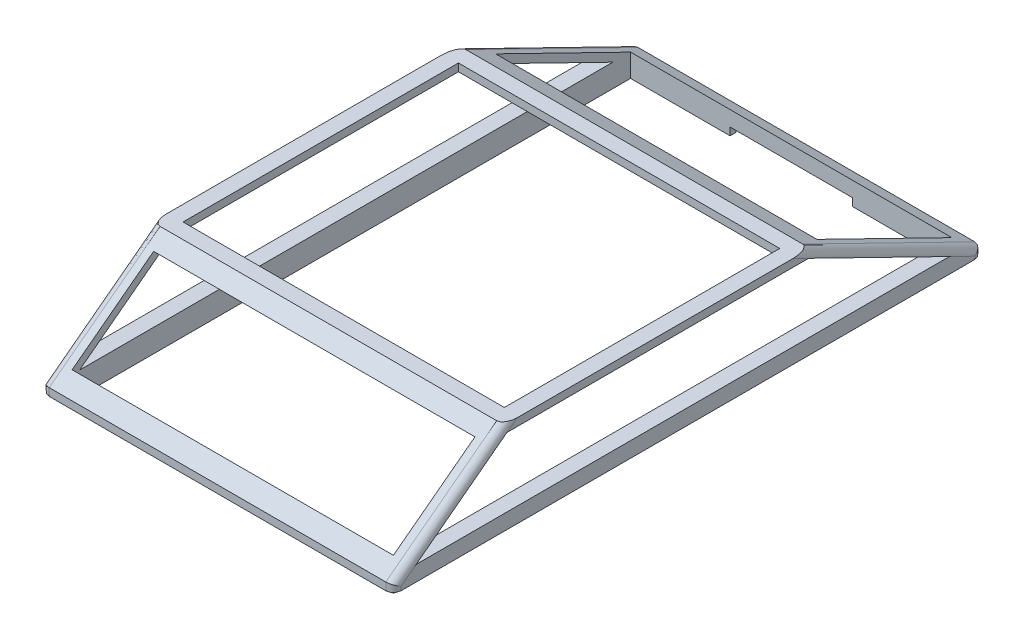
# Autodesk Inventor part: TopLid
Saved by Autodesk Inventor 2023.4 (Build 274418000, 418)
## iProperties
Created: 2026-02-22
Part Number: TopLid
Material: Generic
Document SubType Name: Modeling
Designer: 1017208
Density: 1 g/cm^3
Appearance: Default
Author: 1017208
## iProperties of the stored document TopLid_3DPrint.ipt
Created: 2026-02-22
Part Number: TopLid_3DPrint
Material: Generic
Document SubType Name: Modeling
Designer: 1017208
Density: 1 g/cm^3
Appearance: Default
Author: 1017208
Autodesk Inventor part; units mm, degrees
ref_plane "YZ Plane" through (0, 0, 0) normal (1, 0, 0) x (0, 1, 0)
ref_plane "XZ Plane" through (0, 0, 0) normal (0, 1, 0) x (-1, 0, 0)
ref_plane "XY Plane" through (0, 0, 0) normal (0, 0, 1) x (1, 0, 0)
sketch "Sketch1" plane through (0, 0, 0) normal (0, 1, 0) x (-1, 0, 0)
  line L0 (0, 0) -> (-139.7, 0)
  line L1 (-139.7, 0) -> (-139.7, -238.125)
  line L2 (-139.7, -238.125) -> (0, -238.125)
  line L3 (0, -238.125) -> (0, 0)
  line L4 (-3.175, -3.175) -> (-136.525, -3.175)
  line L5 (-136.525, -3.175) -> (-136.525, -234.95)
  line L6 (-136.525, -234.95) -> (-3.175, -234.95)
  line L7 (-3.175, -234.95) -> (-3.175, -3.175)
  line L8 (0, -238.125) -> (-139.7, -238.125)
  line L9 (-69.85, -238.125) -> (-59.69, -238.125)
  line L10 (-59.69, -238.125) -> (-80.01, -238.125)
  line L11 (-80.01, -234.95) -> (-59.69, -234.95)
  line L12 (-69.85, -238.125) -> (-69.85, -234.95)
  line L13 (-69.85, -238.125) -> (-44.45, -238.125)
  line L14 (-44.45, -238.125) -> (-95.25, -238.125)
  line L15 (-95.25, -238.125) -> (-95.25, -234.95)
  line L16 (-95.25, -234.95) -> (-44.45, -234.95)
  line L17 (-44.45, -234.95) -> (-44.45, -238.125)
  line L18 (-44.45, -238.125) -> (-95.25, -238.125)
  dimension "d0" = 139.7
  dimension "d1" = 238.125
  dimension "d2" = 3.175
  dimension "d45" = 25.4
  dimension "d46" = 50.8
  constraints: 38 end point, 7 parallel, 4 point on line, 3 horizontal, 3 perpendicular, 2 collinear, 2 midpoint, 3 other
  measures "d0" distance of L2.end L1.end
  measures "d1" distance of L1.end L0.end
  measures "d2" distance between parallel lines of L3 L7
  measures "d45" distance of L9.start L13.end
  measures "d46" distance of L15.end L16.end
extrude "Extrusion1" add sketch "Sketch1" along normal blind 3.175 contours L3 L2 L17 L6 L7 L4 L5 L15 L1 L0
sketch "Sketch2" plane through (0, 3.175, 0) normal (0, 1, 0) x (1, 0, 0)
  line L0 (0, 238.125) -> (0, 0) projected
  line L1 (139.7, 238.125) -> (0, 238.125) projected
  line L2 (0, 0) -> (139.7, 0)
  line L3 (139.7, 0) -> (139.7, 238.125)
  line L4 (139.7, 238.125) -> (0, 238.125)
  line L5 (0, 238.125) -> (0, 0)
  line L6 (139.7, -3.175) -> (0, -3.175)
  line L7 (-3.175, 0) -> (-3.175, 238.125)
  line L8 (0, 241.3) -> (139.7, 241.3)
  line L9 (142.875, 238.125) -> (142.875, 0)
  arc A0 (0, 241.3) -> (-3.175, 238.125) centre (0, 238.125) ccw
  arc A1 (-3.175, 0) -> (0, -3.175) centre (0, 0) ccw
  arc A2 (139.7, -3.175) -> (142.875, 0) centre (139.7, 0) ccw
  arc A3 (142.875, 238.125) -> (139.7, 241.3) centre (139.7, 238.125) ccw
  line L10 (136.525, 3.175) -> (3.175, 3.175) projected
  line L11 (139.7, 234.95) -> (3.175, 234.95)
  line L12 (3.175, 234.95) -> (3.175, 3.175)
  line L13 (3.175, 3.175) -> (139.7, 3.175)
  line L14 (139.7, 3.175) -> (139.7, 234.95)
  point P0 (80.01, 238.125)
  point P1 (139.7, 3.175)
  point P2 (139.7, 234.95)
  dimension "d7" = 3.175
  constraints: 24 end point, 8 point on circle, 6 parallel, 4 centre point, 4 coincident, 3 perpendicular, 3 tangent, 2 horizontal
  measures "d7" distance between parallel lines of L2 L6
extrude "Extrusion2" add sketch "Sketch2" along normal blind 3.175 contours L1 L3 L11 L12 L10 L13 L2 L0 | L3 L13 L10 L12 L11 | L6 A1 L7 A0 L8 A3 L9 A2
sketch "Sketch3" plane through (142.875, 3.175, 0) normal (1, 0, 0) x (0, 0, -1)
  line L0 (-3.175, 3.175) -> (241.3, 3.175)
  line L1 (0, 3.175) -> (238.125, 3.175) projected
  line L2 (119.0625, 3.175) -> (119.0625, 38.1)
  line L3 (119.0625, 38.1) -> (42.8625, 38.1)
  line L4 (119.0625, 38.1) -> (169.8625, 38.1)
  line L5 (-3.175, 3.175) -> (42.8625, 38.1)
  line L6 (169.8625, 38.1) -> (241.3, 3.175)
  line L7 (43.9305, 34.925) -> (119.0625, 34.925)
  line L8 (119.0625, 34.925) -> (169.1279, 34.925)
  line L9 (169.1279, 34.925) -> (227.5768, 6.35)
  line L10 (227.5768, 6.35) -> (6.2635, 6.35)
  line L11 (6.2635, 6.35) -> (43.9305, 34.925)
  point P0 (0, -3.175)
  dimension "d10" = 34.925
  dimension "d11" = 76.2
  dimension "d12" = 50.8
  dimension "d13" = 3.175
  constraints: 22 end point, 3 horizontal, 1 midpoint, 1 vertical, 4 other
  measures "d10" distance of L2.start L2.end
  measures "d11" distance of L2.end L3.end
  measures "d12" distance of L2.end L4.end
  measures "d13" distance between parallel lines of L3 L7
extrude "Extrusion3" add sketch "Sketch3" against normal blind 146.05 contours L5 L3 L2 L7 L11 L10 L0 | L2 L10 L9 L8 L4 L6 L0
sketch "Sketch4" plane through (0, 0, 0) normal (0, -1, 0) x (1, 0, 0)
  line L0 (0, 0) -> (139.7, 0) projected
  line L1 (0, -238.125) -> (139.7, -238.125) projected
  line L2 (0, 0) -> (139.7, 0)
  line L3 (139.7, 0) -> (139.7, -238.125)
  line L4 (139.7, -238.125) -> (0, -238.125)
  line L5 (0, -238.125) -> (0, 0)
  line L6 (136.525, -234.95) -> (136.525, -3.175)
  line L7 (136.525, -3.175) -> (3.175, -3.175)
  line L8 (3.175, -3.175) -> (3.175, -234.95)
  line L9 (3.175, -234.95) -> (136.525, -234.95)
  constraints: 16 end point, 4 parallel, 2 perpendicular, 1 horizontal, 3 other
extrude "Extrusion4" cut sketch "Sketch4" against normal blind 36.83 contours L9 L8 L7 L6
sketch "Sketch7" plane through (142.875, 41.275, -42.8625) normal (0, 1, 0) x (1, 0, 0)
  line L0 (-146.05, -36.599) -> (-146.05, 184.7143) projected
  line L1 (-146.05, 0) -> (0, 0)
  line L2 (0, 0) -> (0, 127)
  line L3 (0, 127) -> (-146.05, 127)
  line L4 (-146.05, 127) -> (-146.05, 0)
  line L5 (-139.7, 120.65) -> (-6.35, 120.65)
  line L6 (-6.35, 120.65) -> (-6.35, 6.35)
  line L7 (-6.35, 6.35) -> (-139.7, 6.35)
  line L8 (-139.7, 6.35) -> (-139.7, 120.65)
  point P0 (-142.875, -42.8625)
  dimension "d36" = 6.35
  constraints: 16 end point, 4 parallel, 2 perpendicular, 1 horizontal, 1 point on line, 3 other
  measures "d36" distance between parallel lines of L3 L5
extrude "Extrusion6" cut sketch "Sketch7" against normal blind 36.83 contours L5 L6 L7 L8
fillet "Fillet1" radius 3.175 1 edges at (142.875, 23.8125, -19.8437)
fillet "Fillet2" radius 3.175 1 edges at (142.875, 23.8125, -205.5813)
fillet "Fillet3" radius 3.175 2 edges at (-3.175, 23.8125, -19.8437) (-3.175, 23.8125, -205.5813)
sketch "Sketch8" plane through (0, 0, 0) normal (0, -1, 0) x (1, 0, 0)
  line L0 (0, 0) -> (139.7, 0)
  line L1 (139.7, 0) -> (139.7, -238.125)
  line L2 (139.7, -238.125) -> (0, -238.125)
  line L3 (0, -238.125) -> (0, 0)
  line L4 (0.635, -237.49) -> (139.065, -237.49)
  line L5 (139.065, -237.49) -> (139.065, -0.635)
  line L6 (139.065, -0.635) -> (0.635, -0.635)
  line L7 (0.635, -0.635) -> (0.635, -237.49)
  dimension "d42" = 0.635
  constraints: 16 end point, 4 parallel, 2 perpendicular, 1 horizontal, 3 other
  measures "d42" distance between parallel lines of L2 L4
extrude "Extrusion7" cut sketch "Sketch8" against normal blind 3.175
body "Solid1"
